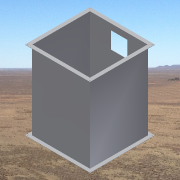
# Autodesk Inventor part: housing
Saved by Autodesk Inventor 2014 SP1 (Build 180222100, 222)
## iProperties
Created: 2014-03-11
Part Number: housing
Material: Aluminum 6061
Document SubType Name: Modeling
Designer: Dave
Density: 2.71 g/cm^3
Appearance: Aluminum - Flat
Mass: 15486.1 g
Surface Area: 45813.7 cm^2
Volume: 5714.43 cm^3
Author: Dave
Autodesk Inventor part; units mm, degrees
ref_plane "YZ Plane" through (0, 0, 0) normal (1, 0, 0) x (0, 1, 0)
ref_plane "XZ Plane" through (0, 0, 0) normal (0, 1, 0) x (-1, 0, 0)
ref_plane "XY Plane" through (0, 0, 0) normal (0, 0, 1) x (1, 0, 0)
sketch "Sketch1" plane through (0, 0, 0) normal (0, 1, 0) x (-1, 0, 0)
  line L0 (0, 0) -> (700, 0)
  line L1 (700, 0) -> (700, 700)
  line L2 (700, 700) -> (0, 700)
  line L3 (0, 700) -> (0, 0)
  dimension "d0" = 700
  dimension "d1" = 700
  constraints: 8 end point, 2 parallel, 1 horizontal, 1 perpendicular
  measures "d0" distance of L0.start L0.end
  measures "d1" distance of L2.end L0.start
extrude "Extrusion1" add sketch "Sketch1" along normal blind 850
sketch "Sketch2" plane through (0, 850, 0) normal (0, 1, 0) x (1, 0, 0)
  line L0 (0, 0) -> (-700, 0) projected
  line L1 (-700, 0) -> (-700, -700) projected
  line L2 (-700, -700) -> (0, -700) projected
  line L3 (0, -700) -> (0, 0) projected
  line L4 (-660, -40) -> (-40, -40)
  line L5 (-40, -40) -> (-40, -660)
  line L6 (-40, -660) -> (-660, -660)
  line L7 (-660, -660) -> (-660, -40)
  dimension "d4" = 40
  constraints: 8 end point, 3 other
  measures "d4" distance between parallel lines of L4 L0
extrude "Extrusion2" cut sketch "Sketch2" against normal blind 1000 contours L4 L5 L6 L7
sketch "Sketch3" plane through (-700, 0, 700) normal (0, 0, 1) x (1, 0, 0)
  line L0 (0, 0) -> (700, 0) projected
  line L1 (700, 0) -> (700, 850) projected
  line L2 (0, 850) -> (700, 850) projected
  line L3 (0, 0) -> (0, 850) projected
  line L4 (0, 2.54) -> (700, 2.54)
  line L5 (700, 2.54) -> (700, 847.46)
  line L6 (700, 847.46) -> (0, 847.46)
  line L7 (0, 847.46) -> (0, 2.54)
  dimension "d7" = 2.54
  dimension "d8" = 2.54
  constraints: 8 end point, 2 parallel, 2 point on line, 1 horizontal, 1 perpendicular
  measures "d7" distance between parallel lines of L6 L2
  measures "d8" distance between parallel lines of L0 L4
extrude "Extrusion3" cut sketch "Sketch3" against normal blind 37.5 contours L3 L6 L1 L4
sketch "Sketch4" plane through (0, 0, 0) normal (0, 0, -1) x (-1, 0, 0)
  line L0 (0, 0) -> (700, 0) projected
  line L1 (700, 0) -> (700, 850) projected
  line L2 (0, 850) -> (700, 850) projected
  line L3 (0, 0) -> (0, 850) projected
  line L4 (0, 2.54) -> (700, 2.54)
  line L5 (700, 2.54) -> (700, 847.46)
  line L6 (700, 847.46) -> (0, 847.46)
  line L7 (0, 847.46) -> (0, 2.54)
  dimension "d11" = 2.54
  dimension "d12" = 2.54
  constraints: 8 end point, 2 parallel, 2 point on line, 1 horizontal, 1 perpendicular
  measures "d11" distance between parallel lines of L6 L2
  measures "d12" distance between parallel lines of L0 L4
extrude "Extrusion4" cut sketch "Sketch4" against normal blind 37.5 contours L3 L6 L1 L4
sketch "Sketch5" plane through (0, 0, 37.5) normal (0, 0, -1) x (-1, 0, 0)
  line L0 (700, 2.54) -> (0, 2.54) projected
  line L1 (0, 847.46) -> (37.5, 847.46)
  line L2 (37.5, 847.46) -> (37.5, 2.54)
  line L3 (37.5, 2.54) -> (0, 2.54)
  line L4 (0, 2.54) -> (0, 847.46)
  line L5 (700, 847.46) -> (662.5, 847.46)
  line L6 (662.5, 847.46) -> (662.5, 2.54)
  line L7 (662.5, 2.54) -> (700, 2.54)
  line L8 (700, 2.54) -> (700, 847.46)
  point P0 (0, 0)
  dimension "d15" = 37.5
  dimension "d16" = 37.5
  constraints: 16 end point, 4 parallel, 2 horizontal, 2 perpendicular, 2 point on line
  measures "d15" distance between parallel lines of L2 L4
  measures "d16" distance between parallel lines of L6 L8
extrude "Extrusion5" cut sketch "Sketch5" against normal blind 1000
sketch "Sketch6" plane through (0, 850, 0) normal (0, 1, 0) x (1, 0, 0)
  line L0 (0, 0) -> (-700, 0) projected
  line L1 (-700, 0) -> (-700, -700) projected
  circle A0 centre (-685, -15) radius 5.0825
  point P0 (-15, -15)
  point P1 (-685, -685)
  point P2 (-15, -685)
  dimension "d19" = 15
  dimension "d20" = 15
  dimension "d23" = 670
  dimension "d26" = 670
  constraints: 1 centre point, 1 horizontal, 1 vertical, 3 other
  measures "d19" distance from line of A0.centre L0
  measures "d20" distance from line of A0.centre L1
  measures "d23" distance of A0.centre point (-15, -15)
  measures "d26" distance of A0.centre point (-685, -685)
hole "Hole1" at (-685, 850, 685) at (-685, 850, 15) at (-15, 850, 15) at (-15, 850, 685) direction (0, -1, 0) diameter 6.35 end through all
sketch "Sketch7" plane through (0, 0, 37.5) normal (0, 0, -1) x (-1, 0, 0)
  line L0 (37.5, 847.46) -> (37.5, 2.54) projected
  line L1 (257.5, 604.8881) -> (437.5, 604.8881)
  line L2 (437.5, 604.8881) -> (437.5, 784.8881)
  line L3 (437.5, 784.8881) -> (257.5, 784.8881)
  line L4 (257.5, 784.8881) -> (257.5, 604.8881)
  point P0 (0, 0)
  dimension "d36" = 220
  dimension "d37" = 180
  dimension "d38" = 180
  constraints: 8 end point, 2 parallel, 1 horizontal, 1 perpendicular
  measures "d36" distance between parallel lines of L4 L0
  measures "d37" distance of L3.end L1.start
  measures "d38" distance of L2.end L3.end
extrude "Extrusion6" cut sketch "Sketch7" against normal blind 10
sketch "Sketch8" plane through (-40, 850, 40) normal (-1, 0, 0) x (0, 0, 1)
  line L0 (620, -850) -> (0, -850) projected
  line L1 (0, 0) -> (0, -850) projected
  line L2 (152.4, -748.4) -> (152.4, -710.3)
  line L3 (152.4, -710.3) -> (190.5, -710.3)
  line L4 (154.94, -748.4) -> (154.94, -712.84)
  line L5 (154.94, -712.84) -> (190.5, -712.84)
  line L6 (154.94, -748.4) -> (152.4, -748.4)
  line L7 (190.5, -710.3) -> (190.5, -712.84)
  line L8 (277.5001, -850) -> (277.5001, -661.936) construction
  line L9 (402.6001, -748.4) -> (402.6001, -710.3)
  line L10 (402.6001, -710.3) -> (364.5001, -710.3)
  line L11 (400.0601, -748.4) -> (400.0601, -712.84)
  line L12 (400.0601, -712.84) -> (364.5001, -712.84)
  line L13 (400.0601, -748.4) -> (402.6001, -748.4)
  line L14 (364.5001, -710.3) -> (364.5001, -712.84)
  point P0 (-40, -850)
  dimension "d41" = 38.1
  dimension "d42" = 38.1
  dimension "d43" = 2.54
  dimension "d44" = 101.6
  dimension "d45" = 152.4
  constraints: 26 end point, 6 symmetric about line, 3 parallel, 3 perpendicular, 1 point on line, 1 other
  measures "d41" distance of L2.start L2.end
  measures "d42" distance of L2.end L3.end
  measures "d43" distance between parallel lines of L4 L2
  measures "d44" distance from line of L4.start L0
  measures "d45" distance between parallel lines of L2 L1
extrude "Extrusion7" add sketch "Sketch8" along normal up to next
body "Solid1"
